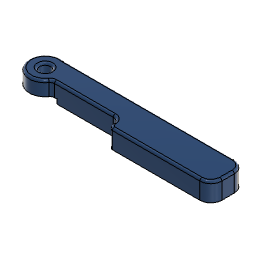
4 inch gate connection bracket - threaded not through (Autodesk Fusion 360 design; units mm, degrees)
Autodesk Fusion 360 part; units mm, degrees
sketch "Main Body" plane through (0, 0, 0) normal (0, 0, 1) x (1, 0, 0)
  line L0 (123.9438, 6.7249) -> (123.9438, 13.8361)
  arc A0 (117.5938, 0.3749) -> (123.9438, 6.7249) centre (117.5938, 6.7249) ccw
  line L1 (123.9438, 6.7249) -> (64.5078, 6.7249) construction
  line L2 (117.5938, 0.3749) -> (67.3042, 0.3749)
  line L3 (61.0843, 7.1711) -> (27.4293, 7.1711)
  arc A1 (65.0438, 3.571) -> (61.0843, 7.1711) centre (61.0843, 3.1937) ccw
  arc A2 (65.0438, 3.571) -> (67.3042, 0.3749) centre (68.2411, 3.4349) ccw
  circle A3 centre (17.8824, 11.2984) radius 3.175
  line L4 (117.5938, 20.1861) -> (19.8575, 20.1861)
  arc A4 (19.8575, 20.1861) -> (25.3469, 6.0854) centre (17.8824, 11.2984) ccw
  arc A5 (27.4293, 7.1711) -> (25.3469, 6.0854) centre (27.4293, 4.6311) ccw
  arc A6 (123.9438, 13.8361) -> (117.5938, 20.1861) centre (117.5938, 13.8361) ccw
  point P0 (123.9438, 8.0934)
  dimension "d173" = 6.35
  dimension "d175" = 59.436
  dimension "d178" = 6.35
  dimension "d221" = 2.54
  dimension "d223" = 50.2896
  dimension "d229" = 6.35
  dimension "d230" = 33.655
  constraint vertical L0
  constraint coincident P0 L0
  constraint tangent L0 A0
  constraint perpendicular L0 L1
  constraint tangent A0 L2
  constraint parallel L1 L2
  constraint tangent L3 A1
  constraint horizontal L3
  constraint concentric A3 A4
  constraint tangent L3 A5
  constraint tangent A4 A5
  constraint perpendicular L0 L4
  constraint tangent L0 A6
  constraint tangent L4 A6
  measures "d173" radius of A0
  measures "d175" distance of L0.start L1.end
  measures "d178" diameter of A3
  measures "d221" radius of A5
  measures "d223" distance of A0.start L2.end
  measures "d229" radius of A6
  measures "d230" distance of L3.start L3.end
extrude "Extrude2" add sketch "Main Body" along normal blind 10.795
ref_plane "WorkPlane2" through (65.2693, 10.7273, 0) normal (0, 0, -1) x (-1, 0, 0)
sketch "Cut out for Actuator" plane through (0, 0, 0) normal (0, 0, -1) x (-1, 0, 0)
  line L0 (-3.356, 0.6564) -> (-28.756, 0.6564)
  line L1 (-28.756, 0.6564) -> (-28.756, 21.8424)
  line L2 (-28.756, 21.8424) -> (-3.356, 21.8424)
  line L3 (-3.356, 21.8424) -> (-3.356, 0.6564)
  dimension "d205" = 25.4
  constraint horizontal L0
  constraint vertical L1
  constraint horizontal L2
  constraint vertical L3
  measures "d205" distance of L0.start L0.end
extrude "Extrude7" cut sketch "Cut out for Actuator" against normal blind 2.54
hole "Hole3" at (109.7706, 10.0261, 0) direction (0, 0, 1) diameter 3.429 depth 8.255 tip angle 180
thread "Thread3" "ANSI Unified Screw Threads 0.164(#8) 8-32 UNC 2B" major diameter 4.1656 minor diameter 3.4163 pitch 0.7937 angle 60 modelled right hand crest width 0.2341 on face at (111.0561, 8.8916, 2.7517) crest through (108.0625, 10.0261, 0.1984)
hole "Hole4" at (81.1448, 10.0261, 0) direction (0, 0, 1) diameter 3.429 depth 8.255 tip angle 180
thread "Thread4" "ANSI Unified Screw Threads 0.164(#8) 8-32 UNC 2B" major diameter 4.1656 minor diameter 3.4163 pitch 0.7937 angle 60 modelled right hand crest width 0.2341 on face at (82.1801, 8.6594, 2.7517) crest through (79.4367, 10.0261, 0.1984)
fillet "Fillet1" radius 1.27 1 faces at (100.8306, 6.9786, 10.795)
